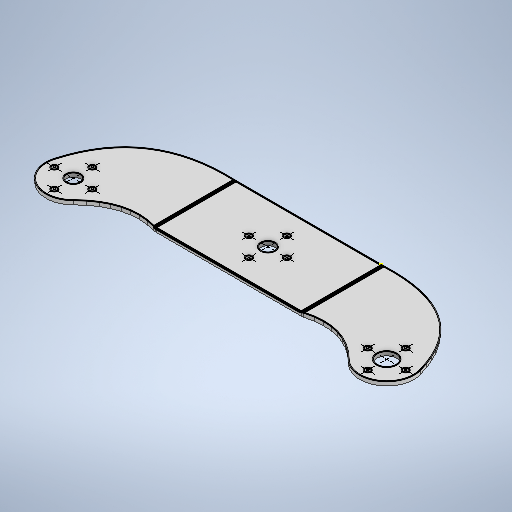
# Autodesk Inventor part: axis_15_bottom_frame
Saved by Autodesk Inventor 2026.1 (Build 301233000, 233)
## iProperties
Created: 2025-08-15
Part Number: axis_15_bottom_frame
Material: Generic
Document SubType Name: Modeling
Designer: LG
Density: 1 g/cm^3
Appearance: Default
Author: LG
Autodesk Inventor part; units mm, degrees
ref_plane "YZ Plane" through (0, 0, 0) normal (1, 0, 0) x (0, 1, 0)
ref_plane "XZ Plane" through (0, 0, 0) normal (0, 1, 0) x (-1, 0, 0)
ref_plane "XY Plane" through (0, 0, 0) normal (0, 0, 1) x (1, 0, 0)
sketch "Sketch1" plane through (0, 0, 0) normal (0, 1, 0) x (-1, 0, 0)
  line L0 (-0.4496, 29.8144) -> (-0.4496, -0.0337)
  line L1 (54.0096, -0.0338) -> (54.0096, 29.8144)
  line L2 (53.5706, 0) -> (53.6221, -0.0838)
  line L3 (53.56, 0) -> (53.5706, 0)
  line L4 (53.56, -0.0837) -> (53.56, 0)
  line L5 (-0.0106, 0) -> (-0.0621, -0.0838)
  line L6 (-0.8993, -0.0972) -> (-0.0106, 0)
  line L7 (53.5706, 0) -> (54.4593, -0.0972)
  line L8 (0, 0) -> (0, -0.0837)
  line L9 (-0.0106, 0) -> (0, 0)
  line L10 (0, 0) -> (53.56, 0)
  line L11 (53.7094, 29.5089) -> (53.5853, 29.9994)
  line L12 (53.56, 29.512) -> (53.7094, 29.5089)
  line L13 (53.56, 30) -> (53.56, 29.512)
  line L14 (-0.1494, 29.5089) -> (-0.0253, 29.9994)
  line L15 (-0.8993, 29.4222) -> (-0.1494, 29.5089)
  line L16 (0, 29.512) -> (0, 30)
  line L17 (-0.1494, 29.5089) -> (0, 29.512)
  line L18 (53.7094, 29.5089) -> (54.4593, 29.4222)
  line L19 (0, 29.512) -> (53.56, 29.512)
  circle A0 centre (26.78, 15) radius 2.6
  circle A1 centre (84.5793, 29) radius 2.6
  circle A2 centre (-31.0193, 29) radius 3.6
  circle A3 centre (91.5793, 29) radius 1.05
  circle A4 centre (84.5793, 36) radius 1.05
  circle A5 centre (84.5793, 22) radius 1.05
  circle A6 centre (77.5793, 29) radius 1.05
  circle A7 centre (-38.0193, 29) radius 1.05
  circle A8 centre (-31.0193, 36) radius 1.05
  circle A9 centre (-31.0193, 22) radius 1.05
  circle A10 centre (-24.0193, 29) radius 1.05
  circle A11 centre (19.78, 15) radius 1.05
  circle A12 centre (26.78, 22) radius 1.05
  circle A13 centre (33.78, 15) radius 1.05
  circle A14 centre (26.78, 8) radius 1.05
  line L20 (53.5853, 29.9994) -> (53.56, 30)
  line L21 (53.6221, -0.0838) -> (53.56, -0.0837)
  line L22 (-0.0621, -0.0838) -> (-0.8993, -0.0972)
  line L23 (-0.0253, 29.9994) -> (-0.8993, 29.4222)
  line L24 (77.602, 36.0383) -> (74.975, 33.6954)
  line L25 (74.975, 33.6954) -> (72.272, 31.7856)
  line L26 (72.272, 31.7856) -> (69.4931, 30.3089)
  line L27 (69.4931, 30.3089) -> (66.6383, 29.2653)
  line L28 (66.6383, 29.2653) -> (63.7075, 28.6549)
  line L29 (63.7075, 28.6549) -> (60.7007, 28.4776)
  line L30 (60.7007, 28.4776) -> (57.618, 28.7333)
  line L31 (57.618, 28.7333) -> (54.4593, 29.4222)
  line L32 (54.4593, -0.0972) -> (53.6221, -0.0838)
  line L33 (-40.5487, 25.8824) -> (-39.4527, 22.5565)
  line L34 (-39.4527, 22.5565) -> (-38.1807, 19.4832)
  line L35 (-38.1807, 19.4832) -> (-36.7234, 16.6331)
  line L36 (-36.7234, 16.6331) -> (-35.0805, 14.0064)
  line L37 (-35.0805, 14.0064) -> (-33.2522, 11.6029)
  line L38 (-33.2522, 11.6029) -> (-31.2384, 9.4228)
  line L39 (-31.2384, 9.4228) -> (-29.0391, 7.4659)
  line L40 (-29.0391, 7.4659) -> (-26.6543, 5.7324)
  line L41 (-26.6543, 5.7324) -> (-24.0841, 4.2221)
  line L42 (-24.0841, 4.2221) -> (-21.3284, 2.9352)
  line L43 (-21.3284, 2.9352) -> (-18.3872, 1.8715)
  line L44 (-18.3872, 1.8715) -> (-15.2606, 1.0312)
  line L45 (-15.2606, 1.0312) -> (-11.9485, 0.4141)
  line L46 (-11.9485, 0.4141) -> (-8.4509, 0.0204)
  line L47 (-8.4509, 0.0204) -> (-4.7678, -0.1501)
  line L48 (-4.7678, -0.1501) -> (-0.8993, -0.0972)
  line L49 (0, 30) -> (-0.0253, 29.9994)
  line L50 (54.4593, -0.0972) -> (58.3278, -0.1501)
  line L51 (58.3278, -0.1501) -> (62.0109, 0.0204)
  line L52 (62.0109, 0.0204) -> (65.5085, 0.4141)
  line L53 (65.5085, 0.4141) -> (68.8206, 1.0312)
  line L54 (68.8206, 1.0312) -> (71.9472, 1.8715)
  line L55 (71.9472, 1.8715) -> (74.8884, 2.9352)
  line L56 (74.8884, 2.9352) -> (77.6441, 4.2221)
  line L57 (77.6441, 4.2221) -> (80.2143, 5.7324)
  line L58 (80.2143, 5.7324) -> (82.5991, 7.4659)
  line L59 (82.5991, 7.4659) -> (84.7984, 9.4228)
  line L60 (84.7984, 9.4228) -> (86.8122, 11.6029)
  line L61 (86.8122, 11.6029) -> (88.6405, 14.0064)
  line L62 (88.6405, 14.0064) -> (90.2834, 16.6331)
  line L63 (90.2834, 16.6331) -> (91.7407, 19.4832)
  line L64 (91.7407, 19.4832) -> (93.0127, 22.5565)
  line L65 (93.0127, 22.5565) -> (94.1087, 25.8824)
  line L66 (54.4593, 29.4222) -> (53.5853, 29.9994)
  line L67 (-0.8993, 29.4222) -> (-4.058, 28.7333)
  line L68 (-4.058, 28.7333) -> (-7.1407, 28.4776)
  line L69 (-7.1407, 28.4776) -> (-10.1475, 28.6549)
  line L70 (-10.1475, 28.6549) -> (-13.0783, 29.2653)
  line L71 (-13.0783, 29.2653) -> (-15.9331, 30.3089)
  line L72 (-15.9331, 30.3089) -> (-18.712, 31.7856)
  line L73 (-18.712, 31.7856) -> (-21.415, 33.6954)
  line L74 (-21.415, 33.6954) -> (-24.042, 36.0383)
  line L75 (0, -0.0837) -> (-0.0621, -0.0838)
  line L76 (53.56, 30) -> (0, 30)
  arc A15 (-24.042, 36.0383) -> (-40.5487, 25.8824) centre (-31.0892, 28.9999) ccw
  arc A16 (94.1087, 25.8824) -> (77.602, 36.0383) centre (84.6492, 28.9999) ccw
  line L77 (53.56, -0.0837) -> (0, -0.0837)
  line L78 (54.4593, 29.4222) -> (54.4593, -0.0972)
  line L79 (-0.8993, -0.0972) -> (-0.8993, 29.4222)
  line L80 (53.56, 0) -> (53.56, 30)
  line L81 (0, 30) -> (0, 0)
  point P0 (0, 0)
  constraints: 164 end point, 17 centre point, 13 equal radius, 10 vertical, 7 parallel, 4 horizontal, 4 perpendicular, 4 point on circle, 2 point on line, 2 tangent, 175 other
extrude "Extrusion1" add sketch "Sketch1" against normal blind 1.5 contours L15 L17 L81 L9 L6 L79 | L79 L48 L47 L46 L45 L44 L43 L42 L41 L40 L39 L38 L37 L36 L35 L34 L33 A15 L74 L73 L72 L71 L70 L69 L68 L67 | L19 L80 L10 L81 | L12 L18 L78 L7 L3 L80 | L31 L30 L29 L28 L27 L26 L25 L24 A16 L65 L64 L63 L62 L61 L60 L59 L58 L57 L56 L55 L54 L53 L52 L51 L50 L78
body "Solid1"
